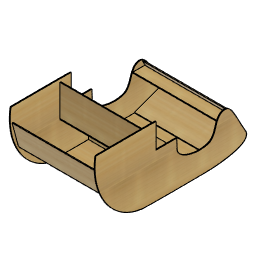
sledi_gs (Autodesk Fusion 360 design; units mm, degrees)
Autodesk Fusion 360 part; units mm, degrees
(part 1 of 2)
sketch "export_vcarve" plane through (0, 0, 0) normal (1, 0, 0) x (0, 1, 0) in component "hlid_1"
  line L0 (2.9518, 787.183) -> (3.1335, 784.5281)
  line L1 (6.7725, 744.8435) -> (7.0756, 742.208)
  line L2 (1.1515, 827.1194) -> (1.2172, 824.451)
  line L3 (5.9084, 752.7581) -> (6.1889, 750.1186)
  line L4 (6.1889, 750.1186) -> (6.4769, 747.4804)
  line L5 (8.7035, 729.0515) -> (9.0515, 726.4246)
  line L6 (11.6958, 708.0792) -> (12.1031, 705.4648)
  line L7 (13.8064, 695.0242) -> (14.2506, 692.4183)
  line L8 (8.363, 731.6799) -> (8.7035, 729.0515)
  line L9 (1.2172, 824.451) -> (1.2907, 821.7834)
  line L10 (7.3862, 739.5739) -> (7.7043, 736.9411)
  line L11 (4.8619, 763.329) -> (5.1122, 760.6844)
  line L12 (2.4528, 795.1537) -> (2.6114, 792.4958)
  line L13 (1.0935, 829.7884) -> (1.1515, 827.1194)
  line L14 (2.6114, 792.4958) -> (2.7778, 789.8389)
  line L15 (1.6626, 811.1211) -> (1.775, 808.4576)
  line L16 (0.9212, 843.1442) -> (0.94, 840.4717)
  line L17 (4.6192, 765.9749) -> (4.8619, 763.329)
  line L18 (14.7021, 689.8142) -> (15.1609, 687.2119)
  line L19 (3.1335, 784.5281) -> (3.3229, 781.8743)
  line L20 (3.5199, 779.2216) -> (3.7245, 776.57)
  line L21 (1.0011, 835.1287) -> (1.0434, 832.4582)
  line L22 (1.2907, 821.7834) -> (1.3721, 819.1166)
  line L23 (6.4769, 747.4804) -> (6.7725, 744.8435)
  line L24 (12.5179, 702.8521) -> (12.94, 700.2411)
  line L25 (0.9248, 853.8401) -> (0.9121, 851.1652)
  line L26 (5.1122, 760.6844) -> (5.37, 758.041)
  line L27 (2.3018, 797.8126) -> (2.4528, 795.1537)
  line L28 (3.9367, 773.9195) -> (4.1566, 771.2701)
  line L29 (5.37, 758.041) -> (5.6354, 755.3989)
  line L30 (12.94, 700.2411) -> (13.3695, 697.6318)
  line L31 (2.023, 803.1333) -> (2.1585, 800.4725)
  line L32 (2.7778, 789.8389) -> (2.9518, 787.183)
  line L33 (1.4612, 816.4506) -> (1.558, 813.7854)
  line L34 (0.94, 840.4717) -> (0.9666, 837.7999)
  line L35 (9.407, 723.7992) -> (9.7699, 721.1753)
  line L36 (1.8951, 805.795) -> (2.023, 803.1333)
  line L37 (48.8864, 554.8424) -> (50.561, 549.8868)
  line L38 (29.6319, 620.2422) -> (30.9452, 615.1513)
  line L39 (10.518, 715.9321) -> (10.9032, 713.3128)
  line L40 (20.1503, 661.291) -> (21.2351, 656.1302)
  line L41 (21.2351, 656.1302) -> (22.3488, 650.9776)
  line L42 (5.6354, 755.3989) -> (5.9084, 752.7581)
  line L43 (83.1421, 467.5368) -> (85.2964, 462.8133)
  line L44 (28.3468, 625.3425) -> (29.6319, 620.2422)
  line L45 (42.4622, 574.7771) -> (44.0269, 569.7769)
  line L46 (47.2391, 559.8094) -> (48.8864, 554.8424)
  line L47 (16.1006, 682.0127) -> (16.5813, 679.4158)
  line L48 (35.0544, 599.9357) -> (36.4802, 594.8834)
  line L49 (8.0299, 734.3098) -> (8.363, 731.6799)
  line L50 (3.3229, 781.8743) -> (3.5199, 779.2216)
  line L51 (40.925, 579.788) -> (42.4622, 574.7771)
  line L52 (50.561, 549.8868) -> (52.2629, 544.9427)
  line L53 (36.4802, 594.8834) -> (37.934, 589.8413)
  line L54 (16.5813, 679.4158) -> (17.0694, 676.8208)
  line L55 (9.0515, 726.4246) -> (9.407, 723.7992)
  line L56 (4.3841, 768.6219) -> (4.6192, 765.9749)
  line L57 (68.795, 500.9914) -> (70.7656, 496.1714)
  line L58 (103.4584, 425.5582) -> (105.8435, 420.9703)
  line L59 (18.0673, 671.6365) -> (19.0943, 666.4598)
  line L60 (0.9666, 837.7999) -> (1.0011, 835.1287)
  line L61 (1.0434, 832.4582) -> (1.0935, 829.7884)
  line L62 (1.775, 808.4576) -> (1.8951, 805.795)
  line L63 (2.1585, 800.4725) -> (2.3018, 797.8126)
  line L64 (7.7043, 736.9411) -> (8.0299, 734.3098)
  line L65 (72.7626, 491.3648) -> (74.786, 486.5716)
  line L66 (15.6271, 684.6114) -> (16.1006, 682.0127)
  line L67 (0.9121, 851.1652) -> (0.9073, 848.491)
  line L68 (11.2958, 710.6952) -> (11.6958, 708.0792)
  line L69 (7.0756, 742.208) -> (7.3862, 739.5739)
  line L70 (70.7656, 496.1714) -> (72.7626, 491.3648)
  line L71 (33.6566, 604.9978) -> (35.0544, 599.9357)
  line L72 (9.7699, 721.1753) -> (10.1402, 718.5529)
  line L73 (3.7245, 776.57) -> (3.9367, 773.9195)
  line L74 (22.3488, 650.9776) -> (23.4912, 645.8333)
  line L75 (81.0139, 472.2745) -> (83.1421, 467.5368)
  line L76 (52.2629, 544.9427) -> (53.992, 540.0103)
  line L77 (63.0428, 515.5293) -> (64.9335, 510.6705)
  line L78 (19.0943, 666.4598) -> (20.1503, 661.291)
  line L79 (96.4554, 439.4155) -> (98.7643, 434.781)
  line L80 (113.1503, 407.3024) -> (115.6362, 402.779)
  line L81 (120.6827, 393.7817) -> (123.2433, 389.3082)
  line L82 (123.2433, 389.3082) -> (125.8287, 384.8517)
  line L83 (59.3417, 525.2849) -> (61.1788, 520.4008)
  line L84 (17.0694, 676.8208) -> (18.0673, 671.6365)
  line L85 (115.6362, 402.779) -> (118.147, 398.272)
  line L86 (212.8912, 261.7857) -> (214.5411, 259.8523)
  line L87 (193.5343, 285.4073) -> (195.116, 283.4096)
  line L88 (53.992, 540.0103) -> (55.7482, 535.0897)
  line L89 (89.6827, 453.4098) -> (91.9145, 448.7301)
  line L90 (209.6083, 265.6688) -> (211.2469, 263.7245)
  line L91 (157.3166, 334.8751) -> (158.758, 332.7574)
  line L92 (39.4156, 584.8094) -> (40.925, 579.788)
  line L93 (27.0902, 630.4519) -> (28.3468, 625.3425)
  line L94 (30.9452, 615.1513) -> (32.2868, 610.0697)
  line L95 (221.1967, 252.1738) -> (222.8746, 250.2681)
  line L96 (222.8746, 250.2681) -> (224.5581, 248.3679)
  line L97 (132.3999, 373.7859) -> (133.7326, 371.5858)
  line L98 (66.851, 505.8244) -> (68.795, 500.9914)
  line L99 (182.6236, 299.5366) -> (184.1649, 297.5027)
  line L100 (98.7643, 434.781) -> (101.0986, 430.1618)
  line L101 (125.8287, 384.8517) -> (128.4387, 380.4124)
  line L102 (110.6896, 411.8423) -> (113.1503, 407.3024)
  line L103 (141.8568, 358.4786) -> (143.2321, 356.3098)
  line L104 (32.2868, 610.0697) -> (33.6566, 604.9978)
  line L105 (85.2964, 462.8133) -> (87.4766, 458.1042)
  line L106 (61.1788, 520.4008) -> (63.0428, 515.5293)
  line L107 (23.4912, 645.8333) -> (24.6623, 640.6974)
  line L108 (101.0986, 430.1618) -> (103.4584, 425.5582)
  line L109 (94.1722, 444.0652) -> (96.4554, 439.4155)
  line L110 (91.9145, 448.7301) -> (94.1722, 444.0652)
  line L111 (201.5001, 275.4714) -> (203.1104, 273.5002)
  line L112 (179.5583, 303.6196) -> (181.088, 301.5756)
  line L113 (136.4163, 367.1989) -> (137.7673, 365.0121)
  line L114 (175.0041, 309.782) -> (176.5164, 307.7228)
  line L115 (76.8357, 481.7921) -> (78.9117, 477.0263)
  line L116 (151.6107, 343.3931) -> (153.0282, 341.2565)
  line L117 (78.9117, 477.0263) -> (81.0139, 472.2745)
  line L118 (64.9335, 510.6705) -> (66.851, 505.8244)
  line L119 (24.6623, 640.6974) -> (25.862, 635.5703)
  line L120 (37.934, 589.8413) -> (39.4156, 584.8094)
  line L121 (211.2469, 263.7245) -> (212.8912, 261.7857)
  line L122 (214.5411, 259.8523) -> (216.1966, 257.9244)
  line L123 (199.8955, 277.448) -> (201.5001, 275.4714)
  line L124 (74.786, 486.5716) -> (76.8357, 481.7921)
  line L125 (181.088, 301.5756) -> (182.6236, 299.5366)
  line L126 (44.0269, 569.7769) -> (45.6193, 564.7876)
  line L127 (188.8236, 291.4317) -> (190.3881, 289.4184)
  line L128 (196.7035, 281.4171) -> (198.2966, 279.4299)
  line L129 (45.6193, 564.7876) -> (47.2391, 559.8094)
  line L130 (153.0282, 341.2565) -> (154.4517, 339.1247)
  line L131 (108.2539, 416.3983) -> (110.6896, 411.8423)
  line L132 (105.8435, 420.9703) -> (108.2539, 416.3983)
  line L133 (25.862, 635.5703) -> (27.0902, 630.4519)
  line L134 (118.147, 398.272) -> (120.6827, 393.7817)
  line L135 (57.5314, 530.1812) -> (59.3417, 525.2849)
  line L136 (87.4766, 458.1042) -> (89.6827, 453.4098)
  line L137 (55.7482, 535.0897) -> (57.5314, 530.1812)
  line L138 (146.0008, 351.9858) -> (147.3943, 349.8307)
  line L139 (131.0734, 375.9904) -> (132.3999, 373.7859)
  line L140 (160.2053, 330.6445) -> (161.6586, 328.5363)
  line L141 (216.1966, 257.9244) -> (217.8577, 256.002)
  line L142 (185.712, 295.4739) -> (187.265, 293.4502)
  line L143 (169.0139, 318.0682) -> (170.5026, 315.9893)
  line L144 (154.4517, 339.1247) -> (155.8811, 336.9975)
  line L145 (219.5244, 254.0851) -> (221.1967, 252.1738)
  line L146 (170.5026, 315.9893) -> (171.9973, 313.9152)
  line L147 (167.531, 320.1521) -> (169.0139, 318.0682)
  line L148 (133.7326, 371.5858) -> (135.0714, 369.3901)
  line L149 (187.265, 293.4502) -> (188.8236, 291.4317)
  line L150 (137.7673, 365.0121) -> (139.1244, 362.8298)
  line L151 (150.1992, 345.5343) -> (151.6107, 343.3931)
  line L152 (171.9973, 313.9152) -> (173.4978, 311.8461)
  line L153 (198.2966, 279.4299) -> (199.8955, 277.448)
  line L154 (190.3881, 289.4184) -> (191.9583, 287.4102)
  line L155 (161.6586, 328.5363) -> (163.1178, 326.433)
  line L156 (207.9753, 267.6186) -> (209.6083, 265.6688)
  line L157 (158.758, 332.7574) -> (160.2053, 330.6445)
  line L158 (173.4978, 311.8461) -> (175.0041, 309.782)
  line L159 (204.7264, 271.5343) -> (206.348, 269.5737)
  line L160 (143.2321, 356.3098) -> (144.6134, 354.1455)
  line L161 (195.116, 283.4096) -> (196.7035, 281.4171)
  line L162 (139.1244, 362.8298) -> (140.4875, 360.6519)
  line L163 (166.054, 322.2409) -> (167.531, 320.1521)
  line L164 (128.4387, 380.4124) -> (129.753, 378.1992)
  line L165 (164.583, 324.3345) -> (166.054, 322.2409)
  line L166 (191.9583, 287.4102) -> (193.5343, 285.4073)
  line L167 (163.1178, 326.433) -> (164.583, 324.3345)
  line L168 (144.6134, 354.1455) -> (146.0008, 351.9858)
  line L169 (206.348, 269.5737) -> (207.9753, 267.6186)
  line L170 (135.0714, 369.3901) -> (136.4163, 367.1989)
  line L171 (140.4875, 360.6519) -> (141.8568, 358.4786)
  line L172 (155.8811, 336.9975) -> (157.3166, 334.8751)
  line L173 (148.7937, 347.6802) -> (150.1992, 345.5343)
  line L174 (176.5164, 307.7228) -> (178.0344, 305.6687)
  line L175 (184.1649, 297.5027) -> (185.712, 295.4739)
  line L176 (178.0344, 305.6687) -> (179.5583, 303.6196)
  line L177 (129.753, 378.1992) -> (131.0734, 375.9904)
  line L178 (203.1104, 273.5002) -> (204.7264, 271.5343)
  line L179 (217.8577, 256.002) -> (219.5244, 254.0851)
  line L180 (305.9355, 168.9723) -> (307.8654, 167.3509)
  line L181 (147.3943, 349.8307) -> (148.7937, 347.6802)
  line L182 (307.8654, 167.3509) -> (309.8006, 165.7362)
  line L183 (262.9865, 208.0195) -> (264.7956, 206.2535)
  line L184 (319.553, 157.7609) -> (321.5187, 156.1857)
  line L185 (294.4641, 178.8362) -> (296.363, 177.1761)
  line L186 (311.7408, 164.1279) -> (313.6862, 162.5263)
  line L187 (313.6862, 162.5263) -> (315.6367, 160.9312)
  line L188 (321.5187, 156.1857) -> (323.4896, 154.6172)
  line L189 (323.4896, 154.6172) -> (325.4655, 153.0554)
  line L190 (250.473, 220.5501) -> (252.2444, 218.7421)
  line L191 (279.4609, 192.3454) -> (281.3179, 190.6348)
  line L192 (325.4655, 153.0554) -> (327.4465, 151.5004)
  line L193 (226.2472, 246.4734) -> (227.9418, 244.5845)
  line L194 (264.7956, 206.2535) -> (266.6101, 204.4935)
  line L195 (300.1765, 173.8752) -> (302.091, 172.2344)
  line L196 (329.4325, 149.952) -> (331.4236, 148.4104)
  line L197 (331.4236, 148.4104) -> (333.4197, 146.8756)
  line L198 (259.3842, 211.5697) -> (261.1827, 209.7916)
  line L199 (231.3476, 240.8236) -> (233.0588, 238.9517)
  line L200 (304.0106, 170.6001) -> (305.9355, 168.9723)
  line L201 (333.4197, 146.8756) -> (335.4208, 145.3475)
  line L202 (335.4208, 145.3475) -> (337.427, 143.8263)
  line L203 (309.8006, 165.7362) -> (311.7408, 164.1279)
  line L204 (288.7986, 183.8548) -> (290.6819, 182.1756)
  line L205 (327.4465, 151.5004) -> (329.4325, 149.952)
  line L206 (337.427, 143.8263) -> (339.4381, 142.3119)
  line L207 (234.7755, 237.0855) -> (236.4978, 235.2251)
  line L208 (266.6101, 204.4935) -> (268.43, 202.7396)
  line L209 (281.3179, 190.6348) -> (283.1802, 188.9303)
  line L210 (317.5923, 159.3427) -> (319.553, 157.7609)
  line L211 (224.5581, 248.3679) -> (226.2472, 246.4734)
  line L212 (236.4978, 235.2251) -> (238.2255, 233.3704)
  line L213 (227.9418, 244.5845) -> (229.6419, 242.7012)
  line L214 (257.5912, 213.3539) -> (259.3842, 211.5697)
  line L215 (285.0478, 187.2322) -> (286.9206, 185.5403)
  line L216 (255.8035, 215.144) -> (257.5912, 213.3539)
  line L217 (315.6367, 160.9312) -> (317.5923, 159.3427)
  line L218 (286.9206, 185.5403) -> (288.7986, 183.8548)
  line L219 (292.5704, 180.5027) -> (294.4641, 178.8362)
  line L220 (252.2444, 218.7421) -> (254.0213, 216.9401)
  line L221 (372.2895, 119.0274) -> (374.3843, 117.6322)
  line L222 (428.303, 85.1437) -> (430.5206, 83.9421)
  line L223 (368.1145, 121.8392) -> (370.1996, 120.4297)
  line L224 (339.4381, 142.3119) -> (341.4543, 140.8044)
  line L225 (283.1802, 188.9303) -> (285.0478, 187.2322)
  line L226 (277.6092, 194.0623) -> (279.4609, 192.3454)
  line L227 (366.0342, 123.2558) -> (368.1145, 121.8392)
  line L228 (272.0857, 199.2503) -> (273.9216, 197.5148)
  line L229 (302.091, 172.2344) -> (304.0106, 170.6001)
  line L230 (389.1829, 108.0687) -> (391.3162, 106.7317)
  line L231 (478.1386, 60.5221) -> (480.4553, 59.4949)
  line L232 (238.2255, 233.3704) -> (239.9588, 231.5214)
  line L233 (395.597, 104.0797) -> (397.7445, 102.7648)
  line L234 (380.6978, 113.49) -> (382.8119, 112.1238)
  line L235 (397.7445, 102.7648) -> (399.8968, 101.4573)
  line L236 (471.2151, 63.6525) -> (473.5185, 62.6009)
  line L237 (233.0588, 238.9517) -> (234.7755, 237.0855)
  line L238 (399.8968, 101.4573) -> (402.0538, 100.1572)
  line L239 (432.7429, 82.7483) -> (434.9697, 81.5621)
  line L240 (378.5885, 114.8635) -> (380.6978, 113.49)
  line L241 (412.9093, 93.7692) -> (415.0945, 92.5141)
  line L242 (391.3162, 106.7317) -> (393.4542, 105.402)
  line L243 (341.4543, 140.8044) -> (343.4754, 139.3037)
  line L244 (384.9308, 110.7648) -> (387.0545, 109.4131)
  line L245 (439.437, 79.2132) -> (441.6775, 78.0504)
  line L246 (268.43, 202.7396) -> (270.2552, 200.9919)
  line L247 (290.6819, 182.1756) -> (292.5704, 180.5027)
  line L248 (353.6555, 131.9042) -> (355.7064, 130.4452)
  line L249 (402.0538, 100.1572) -> (404.2155, 98.8646)
  line L250 (245.1913, 226.0094) -> (246.9465, 224.1838)
  line L251 (239.9588, 231.5214) -> (241.6975, 229.6783)
  line L252 (421.6779, 88.7946) -> (423.8816, 87.57)
  line L253 (273.9216, 197.5148) -> (275.7627, 195.7855)
  line L254 (363.9589, 124.6795) -> (366.0342, 123.2558)
  line L255 (406.3819, 97.5795) -> (408.553, 96.3019)
  line L256 (441.6775, 78.0504) -> (443.9226, 76.8954)
  line L257 (455.2159, 71.2384) -> (457.4881, 70.1307)
  line L258 (448.4263, 74.6089) -> (450.685, 73.4775)
  line L259 (349.5686, 134.8432) -> (351.6096, 133.3702)
  line L260 (351.6096, 133.3702) -> (353.6555, 131.9042)
  line L261 (443.9226, 76.8954) -> (446.1722, 75.7482)
  line L262 (408.553, 96.3019) -> (410.7288, 95.0317)
  line L263 (426.09, 86.353) -> (428.303, 85.1437)
  line L264 (248.707, 222.364) -> (250.473, 220.5501)
  line L265 (254.0213, 216.9401) -> (255.8035, 215.144)
  line L266 (246.9465, 224.1838) -> (248.707, 222.364)
  line L267 (229.6419, 242.7012) -> (231.3476, 240.8236)
  line L268 (270.2552, 200.9919) -> (272.0857, 199.2503)
  line L269 (376.484, 116.2443) -> (378.5885, 114.8635)
  line L270 (446.1722, 75.7482) -> (448.4263, 74.6089)
  line L271 (450.685, 73.4775) -> (452.9482, 72.354)
  line L272 (275.7627, 195.7855) -> (277.6092, 194.0623)
  line L273 (243.4417, 227.8409) -> (245.1913, 226.0094)
  line L274 (241.6975, 229.6783) -> (243.4417, 227.8409)
  line L275 (298.2672, 175.5225) -> (300.1765, 173.8752)
  line L276 (261.1827, 209.7916) -> (262.9865, 208.0195)
  line L277 (347.5326, 136.3231) -> (349.5686, 134.8432)
  line L278 (343.4754, 139.3037) -> (345.5015, 137.8099)
  line L279 (459.7647, 69.031) -> (462.0459, 67.9393)
  line L280 (473.5185, 62.6009) -> (475.8264, 61.5575)
  line L281 (296.363, 177.1761) -> (298.2672, 175.5225)
  line L282 (437.201, 80.3838) -> (439.437, 79.2132)
  line L283 (423.8816, 87.57) -> (426.09, 86.353)
  line L284 (457.4881, 70.1307) -> (459.7647, 69.031)
  line L285 (419.4788, 90.0268) -> (421.6779, 88.7946)
  line L286 (464.3315, 66.8555) -> (466.6216, 65.7798)
  line L287 (574.1431, 25.9943) -> (576.6284, 25.309)
  line L288 (619.4877, 15.046) -> (622.0441, 14.525)
  line L289 (415.0945, 92.5141) -> (417.2843, 91.2667)
  line L290 (466.6216, 65.7798) -> (468.9161, 64.7121)
  line L291 (475.8264, 61.5575) -> (478.1386, 60.5221)
  line L292 (452.9482, 72.354) -> (455.2159, 71.2384)
  line L293 (361.8884, 126.1104) -> (363.9589, 124.6795)
  line L294 (594.1379, 20.7639) -> (596.6552, 20.1508)
  line L295 (417.2843, 91.2667) -> (419.4788, 90.0268)
  line L296 (410.7288, 95.0317) -> (412.9093, 93.7692)
  line L297 (520.5036, 43.2968) -> (522.898, 42.4194)
  line L298 (382.8119, 112.1238) -> (384.9308, 110.7648)
  line L299 (564.2422, 28.8246) -> (566.7114, 28.1037)
  line L300 (357.7621, 128.9932) -> (359.8228, 127.5483)
  line L301 (404.2155, 98.8646) -> (406.3819, 97.5795)
  line L302 (434.9697, 81.5621) -> (437.201, 80.3838)
  line L303 (489.7658, 55.4678) -> (492.1043, 54.4816)
  line L304 (370.1996, 120.4297) -> (372.2895, 119.0274)
  line L305 (430.5206, 83.9421) -> (432.7429, 82.7483)
  line L306 (599.1765, 19.5469) -> (601.7017, 18.9521)
  line L307 (624.6044, 14.0134) -> (627.1685, 13.5111)
  line L308 (569.1845, 27.3917) -> (571.6618, 26.6885)
  line L309 (374.3843, 117.6322) -> (376.484, 116.2443)
  line L310 (462.0459, 67.9393) -> (464.3315, 66.8555)
  line L311 (480.4553, 59.4949) -> (482.7763, 58.4759)
  line L312 (591.6246, 21.386) -> (594.1379, 20.7639)
  line L313 (611.8417, 16.6646) -> (614.3865, 16.1158)
  line L314 (576.6284, 25.309) -> (579.1178, 24.6326)
  line L315 (496.7945, 52.534) -> (499.146, 51.5726)
  line L316 (468.9161, 64.7121) -> (471.2151, 63.6525)
  line L317 (525.2966, 41.5506) -> (527.6994, 40.6904)
  line L318 (616.9351, 15.5763) -> (619.4877, 15.046)
  line L319 (359.8228, 127.5483) -> (361.8884, 126.1104)
  line L320 (561.7772, 29.5544) -> (564.2422, 28.8246)
  line L321 (554.4066, 31.7967) -> (556.8593, 31.0405)
  line L322 (355.7064, 130.4452) -> (357.7621, 128.9932)
  line L323 (387.0545, 109.4131) -> (389.1829, 108.0687)
  line L324 (393.4542, 105.402) -> (395.597, 104.0797)
  line L325 (609.3008, 17.2227) -> (611.8417, 16.6646)
  line L326 (547.073, 34.1181) -> (549.5134, 33.3355)
  line L327 (487.4316, 56.4623) -> (489.7658, 55.4678)
  line L328 (513.3459, 45.9796) -> (515.7276, 45.0769)
  line L329 (566.7114, 28.1037) -> (569.1845, 27.3917)
  line L330 (345.5015, 137.8099) -> (347.5326, 136.3231)
  line L331 (532.5177, 38.9956) -> (534.9332, 38.161)
  line L332 (544.6367, 34.9093) -> (547.073, 34.1181)
  line L333 (482.7763, 58.4759) -> (485.1018, 57.465)
  line L334 (549.5134, 33.3355) -> (551.9579, 32.5618)
  line L335 (522.898, 42.4194) -> (525.2966, 41.5506)
  line L336 (601.7017, 18.9521) -> (604.2308, 18.3664)
  line L337 (534.9332, 38.161) -> (537.3528, 37.3351)
  line L338 (604.2308, 18.3664) -> (606.7639, 17.79)
  line L339 (537.3528, 37.3351) -> (539.7766, 36.5178)
  line L340 (586.6099, 22.6576) -> (589.1153, 22.0173)
  line L341 (632.3083, 12.5346) -> (634.884, 12.0604)
  line L342 (596.6552, 20.1508) -> (599.1765, 19.5469)
  line L343 (506.2267, 48.7384) -> (508.5955, 47.8104)
  line L344 (579.1178, 24.6326) -> (581.6111, 23.9653)
  line L345 (606.7639, 17.79) -> (609.3008, 17.2227)
  line L346 (530.1065, 39.8387) -> (532.5177, 38.9956)
  line L347 (508.5955, 47.8104) -> (510.9686, 46.8908)
  line L348 (539.7766, 36.5178) -> (542.2046, 35.7092)
  line L349 (629.7365, 13.0181) -> (632.3083, 12.5346)
  line L350 (510.9686, 46.8908) -> (513.3459, 45.9796)
  line L351 (622.0441, 14.525) -> (624.6044, 14.0134)
  line L352 (485.1018, 57.465) -> (487.4316, 56.4623)
  line L353 (501.5019, 50.6195) -> (503.8622, 49.6748)
  line L354 (634.884, 12.0604) -> (637.4634, 11.5956)
  line L355 (515.7276, 45.0769) -> (518.1135, 44.1826)
  line L356 (499.146, 51.5726) -> (501.5019, 50.6195)
  line L357 (492.1043, 54.4816) -> (494.4472, 53.5037)
  line L358 (518.1135, 44.1826) -> (520.5036, 43.2968)
  line L359 (527.6994, 40.6904) -> (530.1065, 39.8387)
  line L360 (542.2046, 35.7092) -> (544.6367, 34.9093)
  line L361 (614.3865, 16.1158) -> (616.9351, 15.5763)
  line L362 (581.6111, 23.9653) -> (584.1085, 23.3069)
  line L363 (503.8622, 49.6748) -> (506.2267, 48.7384)
  line L364 (494.4472, 53.5037) -> (496.7945, 52.534)
  line L365 (551.9579, 32.5618) -> (554.4066, 31.7967)
  line L366 (589.1153, 22.0173) -> (591.6246, 21.386)
  line L367 (627.1685, 13.5111) -> (629.7365, 13.0181)
  line L368 (559.3162, 30.293) -> (561.7772, 29.5544)
  line L369 (637.4634, 11.5956) -> (640.0467, 11.1403)
  line L370 (584.1085, 23.3069) -> (586.6099, 22.6576)
  line L371 (556.8593, 31.0405) -> (559.3162, 30.293)
  line L372 (1022.1424, 0.9057) -> (1035.757, 0.9047)
  line L373 (571.6618, 26.6885) -> (574.1431, 25.9943)
  line L374 (736.31, 3.7954) -> (749.9167, 3.5032)
  line L375 (749.9167, 3.5032) -> (763.5239, 3.2291)
  line L376 (1335.2968, 2.4026) -> (1389.7546, 2.7834)
  line L377 (1171.9108, 1.3207) -> (1199.1423, 1.4744)
  line L378 (763.5239, 3.2291) -> (777.1316, 2.9729)
  line L379 (650.4176, 9.4139) -> (653.0197, 9.0061)
  line L380 (1035.757, 0.9047) -> (1049.3718, 0.9127)
  line L381 (1444.2084, 3.1278) -> (1471.4335, 3.2776)
  line L382 (777.1316, 2.9729) -> (790.7399, 2.734)
  line L383 (676.6069, 5.7684) -> (679.2461, 5.4571)
  line L384 (679.2461, 5.4571) -> (681.889, 5.1556)
  line L385 (940.4598, 1.127) -> (954.0729, 1.0623)
  line L386 (899.6224, 1.3954) -> (913.2346, 1.293)
  line L387 (647.8192, 9.8312) -> (650.4176, 9.4139)
  line L388 (1117.448, 1.0734) -> (1144.6793, 1.1859)
  line L389 (858.7883, 1.7846) -> (872.3993, 1.6407)
  line L390 (967.6863, 1.0094) -> (981.2999, 0.9677)
  line L391 (681.889, 5.1556) -> (695.4934, 4.786)
  line L392 (1525.8793, 3.5149) -> (1553.0999, 3.5955)
  line L393 (790.7399, 2.734) -> (804.3487, 2.512)
  line L394 (645.2246, 10.2581) -> (647.8192, 9.8312)
  line L395 (1076.6019, 0.9541) -> (1090.2172, 0.9867)
  line L396 (817.9579, 2.3065) -> (831.5676, 2.1171)
  line L397 (1389.7546, 2.7834) -> (1416.982, 2.9619)
  line L398 (1062.9868, 0.9293) -> (1076.6019, 0.9541)
  line L399 (1049.3718, 0.9127) -> (1062.9868, 0.9293)
  line L400 (1553.0999, 3.5955) -> (1557.9258, 3.6128)
  line L401 (1562.8616, 3.6451) -> (1567.9047, 3.6928)
  line L402 (1567.9047, 3.6928) -> (1573.0523, 3.7562)
  line L403 (1557.9258, 3.6128) -> (1562.8616, 3.6451)
  line L404 (886.0107, 1.5111) -> (899.6224, 1.3954)
  line L405 (926.847, 1.2037) -> (940.4598, 1.127)
  line L406 (1416.982, 2.9619) -> (1444.2084, 3.1278)
  line L407 (653.0197, 9.0061) -> (655.6257, 8.6078)
  line L408 (709.0983, 4.4364) -> (722.7039, 4.1064)
  line L409 (663.4658, 7.4707) -> (666.0866, 7.1108)
  line L410 (671.3394, 6.4202) -> (673.9713, 6.0895)
  line L411 (994.9139, 0.9368) -> (1008.528, 0.9163)
  line L412 (1090.2172, 0.9867) -> (1117.448, 1.0734)
  line L413 (872.3993, 1.6407) -> (886.0107, 1.5111)
  line L414 (1471.4335, 3.2776) -> (1498.6572, 3.4078)
  line L415 (845.1778, 1.9433) -> (858.7883, 1.7846)
  line L416 (954.0729, 1.0623) -> (967.6863, 1.0094)
  line L417 (642.6337, 10.6945) -> (645.2246, 10.2581)
  line L418 (1199.1423, 1.4744) -> (1226.3739, 1.6433)
  line L419 (668.7111, 6.7607) -> (671.3394, 6.4202)
  line L420 (1008.528, 0.9163) -> (1022.1424, 0.9057)
  line L421 (658.2353, 8.2192) -> (660.8487, 7.8401)
  line L422 (660.8487, 7.8401) -> (663.4658, 7.4707)
  line L423 (655.6257, 8.6078) -> (658.2353, 8.2192)
  line L424 (1226.3739, 1.6433) -> (1280.8362, 2.0132)
  line L425 (640.0467, 11.1403) -> (642.6337, 10.6945)
  line L426 (1144.6793, 1.1859) -> (1171.9108, 1.3207)
  line L427 (1498.6572, 3.4078) -> (1525.8793, 3.5149)
  line L428 (695.4934, 4.786) -> (709.0983, 4.4364)
  line L429 (831.5676, 2.1171) -> (845.1778, 1.9433)
  line L430 (673.9713, 6.0895) -> (676.6069, 5.7684)
  line L431 (913.2346, 1.293) -> (926.847, 1.2037)
  line L432 (804.3487, 2.512) -> (817.9579, 2.3065)
  line L433 (722.7039, 4.1064) -> (736.31, 3.7954)
  line L434 (1648.2641, 6.1568) -> (1654.5937, 6.474)
  line L435 (1900.9941, 33.47) -> (1904.4684, 34.1047)
  line L436 (1851.697, 25.407) -> (1855.2488, 25.9332)
  line L437 (1667.4432, 7.1706) -> (1673.9578, 7.5505)
  line L438 (1865.8825, 27.5569) -> (1869.4188, 28.1133)
  line L439 (1605.983, 4.4845) -> (1611.7873, 4.6669)
  line L440 (1714.1332, 10.2935) -> (1720.9854, 10.831)
  line L441 (1762.7926, 14.5667) -> (1769.8511, 15.2776)
  line L442 (981.2999, 0.9677) -> (994.9139, 0.9368)
  line L443 (1833.8996, 22.8868) -> (1841.025, 23.8729)
  line L444 (1617.6746, 4.8675) -> (1623.6424, 5.0869)
  line L445 (1755.7555, 13.8816) -> (1762.7926, 14.5667)
  line L446 (1883.5138, 30.4158) -> (1887.0233, 31.0108)
  line L447 (1707.3211, 9.7796) -> (1714.1332, 10.2935)
  line L448 (1819.6355, 21.0013) -> (1826.7689, 21.9297)
  line L449 (1784.0217, 16.7778) -> (1791.1284, 17.5678)
  line L450 (1720.9854, 10.831) -> (1727.8751, 11.3922)
  line L451 (1887.0233, 31.0108) -> (1890.5264, 31.6137)
  line L452 (1904.4684, 34.1047) -> (1907.9346, 34.7474)
  line L453 (1693.8284, 8.8207) -> (1700.552, 9.2887)
  line L454 (1776.9284, 16.0145) -> (1784.0217, 16.7778)
  line L455 (1687.1531, 8.3753) -> (1693.8284, 8.8207)
  line L456 (1914.8416, 36.0573) -> (1918.2816, 36.7245)
  line L457 (1879.9983, 29.8285) -> (1883.5138, 30.4158)
  line L458 (1805.3713, 19.2292) -> (1812.5021, 20.1013)
  line L459 (1673.9578, 7.5505) -> (1680.5286, 7.9519)
  line L460 (1869.4188, 28.1133) -> (1872.9505, 28.6773)
  line L461 (1727.8751, 11.3922) -> (1734.7997, 11.9776)
  line L462 (1573.0523, 3.7562) -> (1578.3017, 3.8356)
  line L463 (1635.8085, 5.5826) -> (1642.0015, 5.8597)
  line L464 (1858.7971, 26.4669) -> (1862.3419, 27.0081)
  line L465 (1876.4771, 29.2491) -> (1879.9983, 29.8285)
  line L466 (1862.3419, 27.0081) -> (1865.8825, 27.5569)
  line L467 (1642.0015, 5.8597) -> (1648.2641, 6.1568)
  line L468 (1578.3017, 3.8356) -> (1583.6503, 3.9314)
  line L469 (1872.9505, 28.6773) -> (1876.4771, 29.2491)
  line L470 (1583.6503, 3.9314) -> (1589.0954, 4.0438)
  line L471 (1844.5848, 24.3768) -> (1848.1422, 24.8882)
  line L472 (1680.5286, 7.9519) -> (1687.1531, 8.3753)
  line L473 (1848.1422, 24.8882) -> (1851.697, 25.407)
  line L474 (1894.0228, 32.2245) -> (1897.5121, 32.8433)
  line L475 (1826.7689, 21.9297) -> (1833.8996, 22.8868)
  line L476 (1660.9876, 6.8119) -> (1667.4432, 7.1706)
  line L477 (1748.7426, 13.222) -> (1755.7555, 13.8816)
  line L478 (1611.7873, 4.6669) -> (1617.6746, 4.8675)
  line L479 (1918.2816, 36.7245) -> (1921.7123, 37.3999)
  line L480 (1589.0954, 4.0438) -> (1594.6344, 4.1733)
  line L481 (1741.7564, 12.5874) -> (1748.7426, 13.222)
  line L482 (1700.552, 9.2887) -> (1707.3211, 9.7796)
  line L483 (1907.9346, 34.7474) -> (1911.3925, 35.3983)
  line L484 (1280.8362, 2.0132) -> (1335.2968, 2.4026)
  line L485 (1911.3925, 35.3983) -> (1914.8416, 36.0573)
  line L486 (1654.5937, 6.474) -> (1660.9876, 6.8119)
  line L487 (1629.6879, 5.3251) -> (1635.8085, 5.5826)
  line L488 (1798.2458, 18.3848) -> (1805.3713, 19.2292)
  line L489 (666.0866, 7.1108) -> (668.7111, 6.7607)
  line L490 (1812.5021, 20.1013) -> (1819.6355, 21.0013)
  line L491 (1897.5121, 32.8433) -> (1900.9941, 33.47)
  line L492 (1928.5442, 38.7754) -> (1931.9447, 39.4757)
  line L493 (1921.7123, 37.3999) -> (1925.1333, 38.0835)
  line L494 (1734.7997, 11.9776) -> (1741.7564, 12.5874)
  line L495 (1855.2488, 25.9332) -> (1858.7971, 26.4669)
  line L496 (1987.8382, 52.6952) -> (1990.9943, 53.5524)
  line L497 (2041.8101, 69.5521) -> (2044.6132, 70.5794)
  line L498 (1791.1284, 17.5678) -> (1798.2458, 18.3848)
  line L499 (1994.1336, 54.4188) -> (1997.2558, 55.2943)
  line L500 (1952.1106, 43.8547) -> (1955.429, 44.6145)
  line L501 (2018.6047, 61.6824) -> (2021.5781, 62.6325)
  line L502 (1978.2726, 50.1776) -> (1981.477, 51.0078)
  line L503 (1958.7343, 45.3829) -> (1962.0261, 46.16)
  line L504 (1981.477, 51.0078) -> (1984.6656, 51.847)
  line L505 (1841.025, 23.8729) -> (1844.5848, 24.3768)
  line L506 (1600.2644, 4.32) -> (1605.983, 4.4845)
  line L507 (2104.2794, 98.2792) -> (2106.4122, 99.5646)
  line L508 (2027.4643, 64.5614) -> (2030.3763, 65.5402)
  line L509 (1890.5264, 31.6137) -> (1894.0228, 32.2245)
  line L510 (1971.8179, 48.544) -> (1975.0528, 49.3564)
  line L511 (2071.3355, 81.4005) -> (2073.8695, 82.5383)
  line L512 (1623.6424, 5.0869) -> (1629.6879, 5.3251)
  line L513 (2073.8695, 82.5383) -> (2076.377, 83.6863)
  line L514 (2047.3935, 71.6166) -> (2050.1507, 72.6637)
  line L515 (1594.6344, 4.1733) -> (1600.2644, 4.32)
  line L516 (1975.0528, 49.3564) -> (1978.2726, 50.1776)
  line L517 (2081.3112, 86.0134) -> (2083.7372, 87.1925)
  line L518 (2060.9416, 76.9515) -> (2063.5781, 78.0485)
  line L519 (2076.377, 83.6863) -> (2078.8577, 84.8447)
  line L520 (2078.8577, 84.8447) -> (2081.3112, 86.0134)
  line L521 (1925.1333, 38.0835) -> (1928.5442, 38.7754)
  line L522 (1938.7131, 40.9014) -> (1942.0804, 41.627)
  line L523 (2033.2673, 66.5286) -> (2036.1368, 67.5267)
  line L524 (1769.8511, 15.2776) -> (1776.9284, 16.0145)
  line L525 (1931.9447, 39.4757) -> (1935.3344, 40.1844)
  line L526 (1955.429, 44.6145) -> (1958.7343, 45.3829)
  line L527 (2030.3763, 65.5402) -> (2033.2673, 66.5286)
  line L528 (1935.3344, 40.1844) -> (1938.7131, 40.9014)
  line L529 (2036.1368, 67.5267) -> (2038.9845, 68.5345)
  line L530 (2090.8471, 90.7927) -> (2093.1598, 92.0138)
  line L531 (2038.9845, 68.5345) -> (2041.8101, 69.5521)
  line L532 (2088.5055, 89.5821) -> (2090.8471, 90.7927)
  line L533 (1997.2558, 55.2943) -> (2000.3607, 56.179)
  line L534 (2058.2802, 75.8645) -> (2060.9416, 76.9515)
  line L535 (2083.7372, 87.1925) -> (2086.1354, 88.3821)
  line L536 (2086.1354, 88.3821) -> (2088.5055, 89.5821)
  line L537 (1984.6656, 51.847) -> (1987.8382, 52.6952)
  line L538 (2050.1507, 72.6637) -> (2052.8845, 73.7206)
  line L539 (2044.6132, 70.5794) -> (2047.3935, 71.6166)
  line L540 (2015.6115, 60.7417) -> (2018.6047, 61.6824)
  line L541 (2021.5781, 62.6325) -> (2024.5314, 63.5922)
  line L542 (1968.5683, 47.7406) -> (1971.8179, 48.544)
  line L543 (2052.8845, 73.7206) -> (2055.5944, 74.7876)
  line L544 (1962.0261, 46.16) -> (1965.3043, 46.9459)
  line L545 (2006.5167, 57.9761) -> (2009.5672, 58.8886)
  line L546 (2063.5781, 78.0485) -> (2066.1895, 79.1557)
  line L547 (2068.7754, 80.273) -> (2071.3355, 81.4005)
  line L548 (1990.9943, 53.5524) -> (1994.1336, 54.4188)
  line L549 (1965.3043, 46.9459) -> (1968.5683, 47.7406)
  line L550 (2099.9217, 95.7409) -> (2102.1158, 97.0047)
  line L551 (1942.0804, 41.627) -> (1945.436, 42.361)
  line L552 (2095.4434, 93.2455) -> (2097.6975, 94.4879)
  line L553 (2009.5672, 58.8886) -> (2012.5989, 59.8105)
  line L554 (2066.1895, 79.1557) -> (2068.7754, 80.273)
  line L555 (2012.5989, 59.8105) -> (2015.6115, 60.7417)
  line L556 (2102.1158, 97.0047) -> (2104.2794, 98.2792)
  line L557 (2097.6975, 94.4879) -> (2099.9217, 95.7409)
  line L558 (2093.1598, 92.0138) -> (2095.4434, 93.2455)
  line L559 (1945.436, 42.361) -> (1948.7795, 43.1036)
  line L560 (2133.6647, 119.4414) -> (2134.4752, 120.169)
  line L561 (2142.7841, 128.3623) -> (2143.4832, 129.1246)
  line L562 (2143.4832, 129.1246) -> (2144.1728, 129.8898)
  line L563 (2003.4477, 57.0729) -> (2006.5167, 57.9761)
  line L564 (2000.3607, 56.179) -> (2003.4477, 57.0729)
  line L565 (2055.5944, 74.7876) -> (2058.2802, 75.8645)
  line L566 (2024.5314, 63.5922) -> (2027.4643, 64.5614)
  line L567 (1948.7795, 43.1036) -> (1952.1106, 43.8547)
  line L568 (2134.4752, 120.169) -> (2135.2766, 120.8994)
  line L569 (2164.2201, 203.0668) -> (2163.9708, 204.0923)
  line L570 (2147.4759, 133.7597) -> (2148.1073, 134.5426)
  line L571 (2146.1838, 132.2029) -> (2146.8347, 132.9798)
  line L572 (2158.6117, 150.8274) -> (2159.0275, 151.6735)
  line L573 (2151.1157, 138.5012) -> (2151.6874, 139.3019)
  line L574 (2127.7414, 114.4281) -> (2128.614, 115.1358)
  line L575 (2148.7288, 135.3284) -> (2149.3405, 136.1171)
  line L576 (2118.5423, 107.5059) -> (2120.4498, 108.868)
  line L577 (2124.164, 111.6256) -> (2125.9699, 113.0213)
  line L578 (2159.0275, 151.6735) -> (2159.4326, 152.5226)
  line L579 (2136.8522, 122.3689) -> (2137.6262, 123.1079)
  line L580 (2145.5231, 131.4289) -> (2146.1838, 132.2029)
  line L581 (2116.6016, 106.1548) -> (2118.5423, 107.5059)
  line L582 (2156.842, 147.4738) -> (2157.3003, 148.3077)
  line L583 (2158.1852, 149.9845) -> (2158.6117, 150.8274)
  line L584 (2153.3417, 141.7219) -> (2153.8727, 142.5345)
  line L585 (2142.0754, 127.603) -> (2142.7841, 128.3623)
  line L586 (2151.6874, 139.3019) -> (2152.249, 140.1055)
  line L587 (2110.5838, 102.1679) -> (2112.622, 103.4859)
  line L588 (2137.6262, 123.1079) -> (2138.391, 123.8499)
  line L589 (2157.3003, 148.3077) -> (2157.748, 149.1445)
  line L590 (2159.4326, 152.5226) -> (2159.827, 153.3748)
  line L591 (2160.2105, 154.23) -> (2160.5832, 155.0884)
  line L592 (2106.4122, 99.5646) -> (2108.5137, 100.8608)
  line L593 (2154.3935, 143.3502) -> (2154.904, 144.1689)
  line L594 (2128.614, 115.1358) -> (2129.4779, 115.8463)
  line L595 (2141.3573, 126.8465) -> (2142.0754, 127.603)
  line L596 (2112.622, 103.4859) -> (2114.6281, 104.8149)
  line L597 (2114.6281, 104.8149) -> (2116.6016, 106.1548)
  line L598 (2126.86, 113.7233) -> (2127.7414, 114.4281)
  line L599 (2148.1073, 134.5426) -> (2148.7288, 135.3284)
  line L600 (2132.8452, 118.7167) -> (2133.6647, 119.4414)
  line L601 (2152.249, 140.1055) -> (2152.8004, 140.9122)
  line L602 (2132.0167, 117.9948) -> (2132.8452, 118.7167)
  line L603 (2108.5137, 100.8608) -> (2110.5838, 102.1679)
  line L604 (2156.3731, 146.643) -> (2156.842, 147.4738)
  line L605 (2144.8527, 130.6579) -> (2145.5231, 131.4289)
  line L606 (2125.9699, 113.0213) -> (2126.86, 113.7233)
  line L607 (2153.8727, 142.5345) -> (2154.3935, 143.3502)
  line L608 (2152.8004, 140.9122) -> (2153.3417, 141.7219)
  line L609 (2149.9422, 136.9088) -> (2150.534, 137.7035)
  line L610 (2155.8938, 145.8153) -> (2156.3731, 146.643)
  line L611 (2139.8929, 125.3424) -> (2140.6298, 126.093)
  line L612 (2159.827, 153.3748) -> (2160.2105, 154.23)
  line L613 (2135.2766, 120.8994) -> (2136.0689, 121.6327)
  line L614 (2150.534, 137.7035) -> (2151.1157, 138.5012)
  line L615 (2155.4041, 144.9906) -> (2155.8938, 145.8153)
  line L616 (2144.1728, 129.8898) -> (2144.8527, 130.6579)
  line L617 (2136.0689, 121.6327) -> (2136.8522, 122.3689)
  line L618 (2122.3238, 110.2412) -> (2124.164, 111.6256)
  line L619 (2154.904, 144.1689) -> (2155.4041, 144.9906)
  line L620 (2157.748, 149.1445) -> (2158.1852, 149.9845)
  line L621 (2131.1793, 117.2758) -> (2132.0167, 117.9948)
  line L622 (2140.6298, 126.093) -> (2141.3573, 126.8465)
  line L623 (2160.7521, 214.5323) -> (2160.3567, 215.595)
  line L624 (2129.4779, 115.8463) -> (2130.333, 116.5596)
  line L625 (2162.5275, 209.2702) -> (2162.1991, 210.3158)
  line L626 (2146.8347, 132.9798) -> (2147.4759, 133.7597)
  line L627 (2138.391, 123.8499) -> (2139.1466, 124.5947)
  line L628 (2139.1466, 124.5947) -> (2139.8929, 125.3424)
  line L629 (2130.333, 116.5596) -> (2131.1793, 117.2758)
  line L630 (2120.4498, 108.868) -> (2122.3238, 110.2412)
  line L631 (2149.3405, 136.1171) -> (2149.9422, 136.9088)
  line L632 (2166.0636, 175.6919) -> (2166.1633, 176.6257)
  line L633 (2166.1633, 176.6257) -> (2166.2511, 177.5627)
  line L634 (2166.52, 185.1747) -> (2166.4989, 186.1408)
  line L635 (2164.4215, 166.5293) -> (2164.6379, 167.4313)
  line L636 (2161.134, 213.4731) -> (2160.7521, 214.5323)
  line L637 (2161.8574, 211.3649) -> (2161.5024, 212.4173)
  line L638 (2166.5101, 182.296) -> (2166.5256, 183.2523)
  line L639 (2161.9645, 158.5526) -> (2162.2823, 159.4264)
  line L640 (2161.2958, 156.8143) -> (2161.6357, 157.6819)
  line L641 (2160.3567, 215.595) -> (2159.9478, 216.661)
  line L642 (2160.945, 155.9498) -> (2161.2958, 156.8143)
  line L643 (2163.4421, 162.9528) -> (2163.7039, 163.8422)
  line L644 (2165.0874, 198.9982) -> (2164.89, 200.0104)
  line L645 (2166.0034, 192.9949) -> (2165.8825, 193.9872)
  line L646 (2163.9708, 204.0923) -> (2163.7085, 205.1212)
  line L647 (2165.0361, 169.2448) -> (2165.2179, 170.1563)
  line L648 (2166.4989, 186.1408) -> (2166.4654, 187.1102)
  line L649 (2162.2823, 159.4264) -> (2162.589, 160.3033)
  line L650 (2165.6935, 172.9098) -> (2165.8287, 173.834)
  line L651 (2162.8846, 161.1834) -> (2163.1689, 162.0665)
  line L652 (2166.1117, 192.0059) -> (2166.0034, 192.9949)
  line L653 (2166.3269, 178.5029) -> (2166.3908, 179.4463)
  line L654 (2160.5832, 155.0884) -> (2160.945, 155.9498)
  line L655 (2166.2511, 177.5627) -> (2166.3269, 178.5029)
  line L656 (2165.952, 174.7614) -> (2166.0636, 175.6919)
  line L657 (2162.1991, 210.3158) -> (2161.8574, 211.3649)
  line L658 (2161.5024, 212.4173) -> (2161.134, 213.4731)
  line L659 (2164.8428, 168.3365) -> (2165.0361, 169.2448)
  line L660 (2162.589, 160.3033) -> (2162.8846, 161.1834)
  line L661 (2163.1689, 162.0665) -> (2163.4421, 162.9528)
  line L662 (2165.3881, 171.0709) -> (2165.5467, 171.9888)
  line L663 (2164.1937, 165.6305) -> (2164.4215, 166.5293)
  line L664 (2166.2074, 191.0202) -> (2166.1117, 192.0059)
  line L665 (2165.272, 197.9894) -> (2165.0874, 198.9982)
  line L666 (2166.2906, 190.0378) -> (2166.2074, 191.0202)
  line L667 (2161.6357, 157.6819) -> (2161.9645, 158.5526)
  line L668 (2163.7039, 163.8422) -> (2163.9545, 164.7348)
  line L669 (2166.3613, 189.0586) -> (2166.2906, 190.0378)
  line L670 (2163.9545, 164.7348) -> (2164.1937, 165.6305)
  line L671 (2165.6027, 195.9817) -> (2165.4438, 196.9839)
  line L672 (2165.4438, 196.9839) -> (2165.272, 197.9894)
  line L673 (2164.89, 200.0104) -> (2164.6797, 201.0259)
  line L674 (2166.4195, 188.0828) -> (2166.3613, 189.0586)
  line L675 (2163.1444, 207.1889) -> (2162.8425, 208.2279)
  line L676 (1995.6289, 517.129) -> (1993.4063, 520.9411)
  line L677 (2151.5307, 234.1844) -> (2150.8853, 235.309)
  line L678 (2149.5517, 237.5688) -> (2148.8633, 238.704)
  line L679 (2166.5256, 183.2523) -> (2166.5289, 184.2119)
  line L680 (2155.1052, 227.5095) -> (2154.5447, 228.6133)
  line L681 (2100.9644, 323.7122) -> (2097.8105, 329.4626)
  line L682 (2165.8287, 173.834) -> (2165.952, 174.7614)
  line L683 (2124.0074, 282.244) -> (2120.6086, 288.2967)
  line L684 (2165.749, 194.9828) -> (2165.6027, 195.9817)
  line L685 (2166.4654, 187.1102) -> (2166.4195, 188.0828)
  line L686 (2152.1618, 233.0632) -> (2151.5307, 234.1844)
  line L687 (2154.5447, 228.6133) -> (2153.9701, 229.7206)
  line L688 (2165.8825, 193.9872) -> (2165.749, 194.9828)
  line L689 (2023.4996, 467.3265) -> (2021.0814, 471.7579)
  line L690 (2110.629, 306.1987) -> (2107.3731, 312.08)
  line L691 (2043.5902, 430.0896) -> (2038.4364, 439.6934)
  line L692 (2153.9701, 229.7206) -> (2153.3815, 230.8313)
  line L693 (2148.8633, 238.704) -> (2145.195, 245.0479)
  line L694 (2094.6897, 335.1689) -> (2088.545, 346.4485)
  line L695 (2002.3799, 505.3765) -> (2000.1151, 509.3464)
  line L696 (2000.1151, 509.3464) -> (1997.865, 513.264)
  line L697 (2145.195, 245.0479) -> (2141.5667, 251.3509)
  line L698 (2159.0892, 218.8032) -> (2158.6394, 219.8795)
  line L699 (2141.5667, 251.3509) -> (2137.9778, 257.6127)
  line L700 (2113.9198, 300.2743) -> (2110.629, 306.1987)
  line L701 (2164.6797, 201.0259) -> (2164.4564, 202.0447)
  line L702 (2104.1517, 317.9179) -> (2100.9644, 323.7122)
  line L703 (2004.6596, 501.3544) -> (2002.3799, 505.3765)
  line L704 (2021.0814, 471.7579) -> (2018.6823, 476.1388)
  line L705 (2162.8425, 208.2279) -> (2162.5275, 209.2702)
  line L706 (2013.9392, 484.7488) -> (2011.5943, 488.9773)
  line L707 (2166.4824, 181.3429) -> (2166.5101, 182.296)
  line L708 (1991.1968, 524.7001) -> (1988.9999, 528.4059)
  line L709 (2155.6517, 226.4092) -> (2155.1052, 227.5095)
  line L710 (2059.6326, 400.1251) -> (2048.8382, 420.2924)
  line L711 (2065.1869, 389.7586) -> (2059.6326, 400.1251)
  line L712 (2038.4364, 439.6934) -> (2033.3726, 449.102)
  line L713 (2165.5467, 171.9888) -> (2165.6935, 172.9098)
  line L714 (2157.6988, 222.0423) -> (2157.2078, 223.1288)
  line L715 (2006.955, 497.2803) -> (2004.6596, 501.3544)
  line L716 (2165.2179, 170.1563) -> (2165.3881, 171.0709)
  line L717 (2166.5289, 184.2119) -> (2166.52, 185.1747)
  line L718 (2164.4564, 202.0447) -> (2164.2201, 203.0668)
  line L719 (2166.3908, 179.4463) -> (2166.4426, 180.393)
  line L720 (2156.703, 224.2188) -> (2156.1843, 225.3123)
  line L721 (2159.9478, 216.661) -> (2159.5253, 217.7304)
  line L722 (2088.545, 346.4485) -> (2082.5264, 357.549)
  line L723 (2150.2256, 236.4372) -> (2149.5517, 237.5688)
  line L724 (2166.4426, 180.393) -> (2166.4824, 181.3429)
  line L725 (2164.6379, 167.4313) -> (2164.8428, 168.3365)
  line L726 (2163.433, 206.1534) -> (2163.1444, 207.1889)
  line L727 (2082.5264, 357.549) -> (2076.6298, 368.4687)
  line L728 (2048.8382, 420.2924) -> (2043.5902, 430.0896)
  line L729 (2097.8105, 329.4626) -> (2094.6897, 335.1689)
  line L730 (2152.7787, 231.9455) -> (2152.1618, 233.0632)
  line L731 (2137.9778, 257.6127) -> (2134.428, 263.8332)
  line L732 (2163.7085, 205.1212) -> (2163.433, 206.1534)
  line L733 (1988.9999, 528.4059) -> (1986.8151, 532.0581)
  line L734 (2156.1843, 225.3123) -> (2155.6517, 226.4092)
  line L735 (2159.5253, 217.7304) -> (2159.0892, 218.8032)
  line L736 (1947.956, 589.696) -> (1946.9311, 590.9852)
  line L737 (2134.428, 263.8332) -> (2130.9166, 270.012)
  line L738 (1909.8968, 627.5207) -> (1908.8497, 628.2547)
  line L739 (2033.3726, 449.102) -> (2028.395, 458.3137)
  line L740 (1973.9312, 552.8353) -> (1971.8168, 556.1067)
  line L741 (1938.7452, 600.7744) -> (1937.7227, 601.932)
  line L742 (1993.4063, 520.9411) -> (1991.1968, 524.7001)
  line L743 (2018.6823, 476.1388) -> (2016.3017, 480.4692)
  line L744 (1955.1504, 580.2679) -> (1954.12, 581.6578)
  line L745 (2153.3815, 230.8313) -> (2152.7787, 231.9455)
  line L746 (1959.2825, 574.5657) -> (1957.2142, 577.4453)
  line L747 (2158.176, 220.9592) -> (2157.6988, 222.0423)
  line L748 (1997.865, 513.264) -> (1995.6289, 517.129)
  line L749 (2016.3017, 480.4692) -> (2013.9392, 484.7488)
  line L750 (1971.8168, 556.1067) -> (1969.7105, 559.3228)
  line L751 (2076.6298, 368.4687) -> (2070.8514, 379.2059)
  line L752 (2009.2663, 493.1546) -> (2006.955, 497.2803)
  line L753 (1911.986, 626.0063) -> (1910.9422, 626.7712)
  line L754 (1954.12, 581.6578) -> (1953.0907, 583.0334)
  line L755 (1952.0622, 584.3947) -> (1951.0346, 585.7416)
  line L756 (1931.5848, 608.5673) -> (1930.5608, 609.6212)
  line L757 (1922.346, 617.5111) -> (1921.3154, 618.4294)
  line L758 (1915.1079, 623.6187) -> (1914.0688, 624.43)
  line L759 (1939.7677, 599.602) -> (1938.7452, 600.7744)
  line L760 (1953.0907, 583.0334) -> (1952.0622, 584.3947)
  line L761 (2150.8853, 235.309) -> (2150.2256, 236.4372)
  line L762 (1969.7105, 559.3228) -> (1967.6118, 562.4834)
  line L763 (1946.9311, 590.9852) -> (1945.9067, 592.2598)
  line L764 (2028.395, 458.3137) -> (2023.4996, 467.3265)
  line L765 (2130.9166, 270.012) -> (2127.4433, 276.149)
  line L766 (1967.6118, 562.4834) -> (1965.5201, 565.5882)
  line L767 (1935.6776, 604.2031) -> (1934.6548, 605.3165)
  line L768 (1950.0077, 587.0742) -> (1948.9815, 588.3923)
  line L769 (1908.8497, 628.2547) -> (1907.8008, 628.9731)
  line L770 (1926.4592, 613.6866) -> (1925.4321, 614.6654)
  line L771 (1927.4855, 612.6928) -> (1926.4592, 613.6866)
  line L772 (1936.7002, 603.075) -> (1935.6776, 604.2031)
  line L773 (1921.3154, 618.4294) -> (1920.2837, 619.3325)
  line L774 (2070.8514, 379.2059) -> (2065.1869, 389.7586)
  line L775 (2158.6394, 219.8795) -> (2158.176, 220.9592)
  line L776 (1916.1457, 622.7921) -> (1915.1079, 623.6187)
  line L777 (1961.356, 571.6296) -> (1959.2825, 574.5657)
  line L778 (1945.9067, 592.2598) -> (1944.8827, 593.52)
  line L779 (1924.4043, 615.6291) -> (1923.3756, 616.5777)
  line L780 (2127.4433, 276.149) -> (2124.0074, 282.244)
  line L781 (2107.3731, 312.08) -> (2104.1517, 317.9179)
  line L782 (2117.2462, 294.3068) -> (2113.9198, 300.2743)
  line L783 (1963.435, 568.637) -> (1961.356, 571.6296)
  line L784 (1942.836, 595.9967) -> (1941.813, 597.2131)
  line L785 (1982.4795, 539.2012) -> (1980.3278, 542.6916)
  line L786 (2011.5943, 488.9773) -> (2009.2663, 493.1546)
  line L787 (1956.1817, 578.8637) -> (1955.1504, 580.2679)
  line L788 (2120.6086, 288.2967) -> (2117.2462, 294.3068)
  line L789 (2157.2078, 223.1288) -> (2156.703, 224.2188)
  line L790 (1978.1862, 546.1275) -> (1976.0542, 549.5089)
  line L791 (1920.2837, 619.3325) -> (1919.251, 620.2203)
  line L792 (1925.4321, 614.6654) -> (1924.4043, 615.6291)
  line L793 (1984.6418, 535.6567) -> (1982.4795, 539.2012)
  line L794 (1933.6318, 606.415) -> (1932.6085, 607.4986)
  line L795 (1923.3756, 616.5777) -> (1922.346, 617.5111)
  line L796 (1943.8592, 594.7656) -> (1942.836, 595.9967)
  line L797 (1928.5112, 611.6839) -> (1927.4855, 612.6928)
  line L798 (1957.2142, 577.4453) -> (1956.1817, 578.8637)
  line L799 (1948.9815, 588.3923) -> (1947.956, 589.696)
  line L800 (1937.7227, 601.932) -> (1936.7002, 603.075)
  line L801 (1917.182, 621.9501) -> (1916.1457, 622.7921)
  line L802 (1951.0346, 585.7416) -> (1950.0077, 587.0742)
  line L803 (1918.2171, 621.0929) -> (1917.182, 621.9501)
  line L804 (1910.9422, 626.7712) -> (1909.8968, 627.5207)
  line L805 (1913.0281, 625.2258) -> (1911.986, 626.0063)
  line L806 (1907.8008, 628.9731) -> (1906.75, 629.676)
  line L807 (1976.0542, 549.5089) -> (1973.9312, 552.8353)
  line L808 (1932.6085, 607.4986) -> (1931.5848, 608.5673)
  line L809 (1930.5608, 609.6212) -> (1929.5363, 610.66)
  line L810 (1980.3278, 542.6916) -> (1978.1862, 546.1275)
  line L811 (1941.813, 597.2131) -> (1940.7903, 598.4148)
  line L812 (1944.8827, 593.52) -> (1943.8592, 594.7656)
  line L813 (1919.251, 620.2203) -> (1918.2171, 621.0929)
  line L814 (1965.5201, 565.5882) -> (1963.435, 568.637)
  line L815 (1929.5363, 610.66) -> (1928.5112, 611.6839)
  line L816 (1914.0688, 624.43) -> (1913.0281, 625.2258)
  line L817 (1940.7903, 598.4148) -> (1939.7677, 599.602)
  line L818 (1934.6548, 605.3165) -> (1933.6318, 606.415)
  line L819 (1986.8151, 532.0581) -> (1984.6418, 535.6567)
  line L820 (1874.0589, 643.3839) -> (1872.92, 643.5902)
  line L821 (1906.75, 629.676) -> (1905.6973, 630.3633)
  line L822 (1881.9292, 641.4807) -> (1880.8154, 641.8016)
  line L823 (1897.1997, 635.2966) -> (1896.127, 635.8423)
  line L824 (1858.9352, 644.774) -> (1857.7414, 644.7641)
  line L825 (1836.6851, 641.9978) -> (1835.3981, 641.6807)
  line L826 (1905.6973, 630.3633) -> (1904.6427, 631.0349)
  line L827 (1884.1468, 640.7904) -> (1883.0397, 641.1437)
  line L828 (1878.5775, 642.3944) -> (1877.4533, 642.6663)
  line L829 (1880.8154, 641.8016) -> (1879.6982, 642.1061)
  line L830 (1877.4533, 642.6663) -> (1876.3255, 642.9219)
  line L831 (1869.4799, 644.1103) -> (1868.3252, 644.2507)
  line L832 (1864.8363, 644.572) -> (1863.6649, 644.6459)
  line L833 (1840.5121, 642.8455) -> (1839.2421, 642.5802)
  line L834 (1863.6649, 644.6459) -> (1862.4891, 644.703)
  line L835 (1902.5272, 632.3312) -> (1901.4663, 632.9558)
  line L836 (1843.0358, 643.3245) -> (1841.7767, 643.0936)
  line L837 (1893.974, 636.8859) -> (1892.8936, 637.3838)
  line L838 (1888.5439, 639.2157) -> (1887.4493, 639.6336)
  line L839 (1861.309, 644.7434) -> (1860.1244, 644.7671)
  line L840 (1885.2508, 640.4209) -> (1884.1468, 640.7904)
  line L841 (1883.0397, 641.1437) -> (1881.9292, 641.4807)
  line L842 (1850.4791, 644.3503) -> (1849.2515, 644.222)
  line L843 (1875.1941, 643.1611) -> (1874.0589, 643.3839)
  line L844 (1901.4663, 632.9558) -> (1900.4031, 633.5647)
  line L845 (1886.3516, 640.0353) -> (1885.2508, 640.4209)
  line L846 (1867.1664, 644.3744) -> (1866.0035, 644.4815)
  line L847 (1841.7767, 643.0936) -> (1840.5121, 642.8455)
  line L848 (1839.2421, 642.5802) -> (1837.9664, 642.2976)
  line L849 (1899.3377, 634.1578) -> (1898.2699, 634.7351)
  line L850 (1896.127, 635.8423) -> (1895.0518, 636.372)
  line L851 (1866.0035, 644.4815) -> (1864.8363, 644.572)
  line L852 (1900.4031, 633.5647) -> (1899.3377, 634.1578)
  line L853 (1856.543, 644.7374) -> (1855.3399, 644.6938)
  line L854 (1813.948, 633.9942) -> (1812.7135, 633.3954)
  line L855 (1895.0518, 636.372) -> (1893.974, 636.8859)
  line L856 (1904.6427, 631.0349) -> (1903.586, 631.6909)
  line L857 (1827.0343, 639.2443) -> (1825.6633, 638.7811)
  line L858 (1862.4891, 644.703) -> (1861.309, 644.7434)
  line L859 (1870.6305, 643.9535) -> (1869.4799, 644.1103)
  line L860 (1812.7135, 633.3954) -> (1811.4921, 632.7837)
  line L861 (1766.0695, 590.152) -> (1765.3536, 589.0293)
  line L862 (1852.9193, 644.5559) -> (1851.7017, 644.4616)
  line L863 (1805.5772, 629.5338) -> (1804.4318, 628.8463)
  line L864 (1788.6643, 617.1178) -> (1787.7024, 616.2461)
  line L865 (1792.6196, 620.4958) -> (1791.6144, 619.6678)
  line L866 (1835.3981, 641.6807) -> (1834.1053, 641.3462)
  line L867 (1787.7024, 616.2461) -> (1786.751, 615.3639)
  line L868 (1854.132, 644.6333) -> (1852.9193, 644.5559)
  line L869 (1855.3399, 644.6938) -> (1854.132, 644.6333)
  line L870 (1879.6982, 642.1061) -> (1878.5775, 642.3944)
  line L871 (1807.9052, 630.8716) -> (1806.7349, 630.2089)
  line L872 (1848.0188, 644.0767) -> (1846.7809, 643.9143)
  line L873 (1857.7414, 644.7641) -> (1856.543, 644.7374)
  line L874 (1799.9721, 625.9744) -> (1798.8871, 625.2265)
  line L875 (1889.6357, 638.7818) -> (1888.5439, 639.2157)
  line L876 (1898.2699, 634.7351) -> (1897.1997, 635.2966)
  line L877 (1784.8794, 613.5679) -> (1783.9589, 612.6544)
  line L878 (1876.3255, 642.9219) -> (1875.1941, 643.1611)
  line L879 (1851.7017, 644.4616) -> (1850.4791, 644.3503)
  line L880 (1837.9664, 642.2976) -> (1836.6851, 641.9978)
  line L881 (1890.7245, 638.3318) -> (1889.6357, 638.7818)
  line L882 (1891.8104, 637.8658) -> (1890.7245, 638.3318)